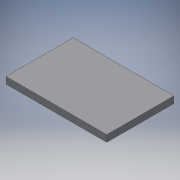
# Autodesk Inventor part: Side wall
Saved by Autodesk Inventor 2016 (Build 200138000, 138)
## iProperties
Created: 2016-04-09
Part Number: Side wall
Material: Generic
Document SubType Name: Modeling
Designer: Vijay
Density: 1 g/cm^3
Appearance: Default
Author: Vijay
Autodesk Inventor part; units mm, degrees
ref_plane "YZ Plane" through (0, 0, 0) normal (1, 0, 0) x (0, 1, 0)
ref_plane "XZ Plane" through (0, 0, 0) normal (0, 1, 0) x (-1, 0, 0)
ref_plane "XY Plane" through (0, 0, 0) normal (0, 0, 1) x (1, 0, 0)
sketch "Sketch1" plane through (0, 0, 0) normal (0, 0, 1) x (1, 0, 0)
  line L0 (-10.6243, -0.0072) -> (4.3757, -0.0072)
  line L1 (4.3757, -0.0072) -> (4.3757, -0.5072)
  line L2 (4.3757, -0.5072) -> (-10.6243, -0.5072)
  line L3 (-10.6243, -0.5072) -> (-10.6243, -0.0072)
  point P0 (0, 0)
  dimension "d0" = 0.5
  dimension "d1" = 15
  constraints: 8 end point, 2 parallel, 1 horizontal, 1 perpendicular
  measures "d0" distance of L2.end L0.start
  measures "d1" distance of L1.end L2.end
extrude "Extrusion1" add sketch "Sketch1" along normal blind 10
sketch "Sketch2" plane through (-10.6243, -0.0072, 0) normal (0, 1, 0) x (1, 0, 0)
  line L0 (0, 0) -> (15, 0) construction
  line L1 (7.5, 0) -> (7.5, -10.8529) construction
  line L2 (15, -5.4265) -> (-1.0951, -5.4265) construction
  line L3 (5.5, 2) -> (9.5, 2)
  line L4 (9.5, 2) -> (9.5, 0)
  line L5 (9.5, 0) -> (5.5, 0)
  line L6 (5.5, 0) -> (5.5, 2)
  point P0 (10.6243, 0)
  dimension "d4" = 4
  dimension "d5" = 2
  constraints: 12 end point, 2 horizontal, 2 parallel, 1 midpoint, 1 perpendicular, 1 point on line, 1 vertical, 1 other
  measures "d4" distance of L3.start L3.end
  measures "d5" distance of L5.end L3.start
extrude "Extrusion2" add sketch "Sketch2" against normal blind 0.5
body "Solid1"
